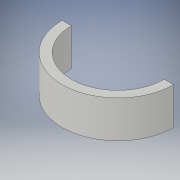
# Autodesk Inventor part: graber base
Saved by Autodesk Inventor 2019 (Build 230136000, 136)
## iProperties
Created: 2020-10-22
Part Number: graber base
Material: Generic
Document SubType Name: Modeling
Designer: User
Density: 1 g/cm^3
Appearance: Default
Author: User
Autodesk Inventor part; units mm, degrees
ref_plane "YZ Plane" through (0, 0, 0) normal (1, 0, 0) x (0, 1, 0)
ref_plane "XZ Plane" through (0, 0, 0) normal (0, 1, 0) x (-1, 0, 0)
ref_plane "XY Plane" through (0, 0, 0) normal (0, 0, 1) x (1, 0, 0)
sketch "Sketch1" plane through (0, 0, 0) normal (0, 1, 0) x (-1, 0, 0)
  arc A0 (31.75, 0) -> (-31.75, 0) centre (0, 0) ccw
  arc A1 (38.1, 0) -> (-38.1, 0) centre (0, 0) ccw
  line L0 (38.1, 0) -> (31.75, 0)
  line L1 (-31.75, 0) -> (-38.1, 0)
  dimension "d0" = 31.75
  dimension "d1" = 38.1
  constraints: 4 end point, 4 point on circle, 2 centre point, 2 coincident, 1 collinear, 1 horizontal
  measures "d0" radius of A0
  measures "d1" radius of A1
extrude "Extrusion1" add sketch "Sketch1" along normal blind 25.4
body "Solid1"
